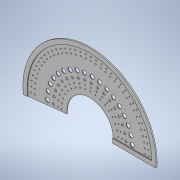
# Autodesk Inventor part: linerCone
Saved by Autodesk Inventor 2021.2 (Build 252289000, 289)
## iProperties
Created: 2021-06-06
Part Number: linerCone
Material: Generic
Document SubType Name: Modeling
Designer: Ryan
Density: 1 g/cm^3
Appearance: Default
Author: Ryan
Autodesk Inventor part; units mm, degrees
ref_plane "YZ Plane" through (0, 0, 0) normal (1, 0, 0) x (0, 1, 0)
ref_plane "XZ Plane" through (0, 0, 0) normal (0, 1, 0) x (-1, 0, 0)
ref_plane "XY Plane" through (0, 0, 0) normal (0, 0, 1) x (1, 0, 0)
sketch "Sketch1" plane through (0, 0, 0) normal (0, 0, 1) x (1, 0, 0)
  arc A0 (33.7972, 0) -> (-33.6117, -3.5367) centre (0, 0) ccw
  line L0 (0, 0) -> (-33.6117, -3.5367) construction
  line L1 (0, 0) -> (33.7972, 0) construction
  arc A1 (90.9472, 0) -> (-90.4486, -9.5105) centre (0, 0) ccw
  line L2 (0, 0) -> (-90.4486, -9.5105) construction
  line L3 (0, 0) -> (90.9472, 0) construction
  line L4 (33.7972, 0) -> (90.9472, 0)
  line L5 (-33.6117, -3.5367) -> (-90.4486, -9.5105)
  dimension "d2" = 33.7972
  dimension "d3" = 186.007
  dimension "d4" = 90.9472
  dimension "d5" = 186.002
  constraints: 12 end point, 4 point on circle, 2 centre point, 2 coincident, 1 collinear
  measures "d2" radius of A0
  measures "d4" radius of A1
extrude "Extrusion1" add sketch "Sketch1" along normal blind 0.7937
sketch "Sketch2" plane through (0, 0, 0.7937) normal (0, 0, 1) x (1, 0, 0)
  arc A0 (97.2972, 0) -> (-96.7638, -10.1743) centre (0, 0) ccw
  line L0 (-90.4486, -9.5105) -> (-33.6117, -3.5367) projected
  line L1 (-33.6117, -3.5367) -> (-96.7638, -10.1743)
  arc A1 (90.9472, 0) -> (-90.4486, -9.5105) centre (0, 0) ccw projected
  line L2 (33.7972, 0) -> (90.9472, 0) projected
  line L3 (33.7972, 0) -> (97.2972, 0)
  arc A2 (33.7972, 0) -> (-33.6117, -3.5367) centre (0, 0) ccw projected
  line L4 (33.7972, 0) -> (97.0898, 0)
  line L5 (97.0898, 0) -> (97.0898, -6.35)
  line L6 (97.0898, -6.35) -> (33.7972, -6.35)
  line L7 (33.7972, -6.35) -> (33.7972, 0)
  dimension "d10" = 97.2972
  dimension "d13" = 6.35
  constraints: 12 end point, 3 point on circle, 2 collinear, 2 parallel, 1 centre point, 1 coincident, 1 horizontal, 1 perpendicular
  measures "d10" radius of A0
  measures "d13" distance of L4.end L5.end
extrude "Extrusion2" add sketch "Sketch2" along normal mid plane 1.5875 contours L3 A1 L1 A0 | L5 L6 L7 L2 L3
sketch "Sketch3" plane through (0, 0, 0.7937) normal (0, 0, 1) x (1, 0, 0)
  circle A0 centre (80.7872, 2.54) radius 0.7938
  circle A1 centre (85.8672, 2.54) radius 0.7937
  line L0 (33.7972, 0) -> (33.7972, -6.35) projected
  line L1 (90.9472, 0) -> (33.7972, 0) projected
  point P0 (0, 0)
  dimension "d14" = 1.5875
  dimension "d15" = 1.5875
  dimension "d18" = 2.54
  dimension "d19" = 2.54
  dimension "d34" = 5.08
  dimension "d35" = 10.16
  constraints: 2 centre point, 1 coincident
  measures "d14" diameter of A0
  measures "d15" diameter of A1
  measures "d18" distance from line of L1 A0.centre
  measures "d19" distance from line of L1 A1.centre
  measures "d34" horizontal distance of point (90.947, 0) A1.centre
  measures "d35" horizontal distance of A0.centre L1.start
extrude "Extrusion3" cut sketch "Sketch3" against normal through all
pattern_circular "Circular Pattern1" count 36 over 180 about axis through (0, 0, 0) along (0, 0, 1) of "Extrusion3"
sketch "Sketch4" plane through (0, 0, 0.7937) normal (0, 0, 1) x (1, 0, 0)
  circle A0 centre (61.7372, 5.08) radius 3.175
  circle A1 centre (52.8472, 5.08) radius 1.5875
  circle A2 centre (46.4972, 5.08) radius 0.7938
  circle A3 centre (41.4172, 5.08) radius 0.7937
  line L0 (90.9472, 0) -> (33.7972, 0) projected
  line L1 (33.7972, 0) -> (33.7972, -6.35) projected
  circle A4 centre (80.7872, 2.54) radius 0.7938 projected
  point P0 (0, 0)
  dimension "d25" = 6.35
  dimension "d26" = 3.175
  dimension "d27" = 1.5875
  dimension "d28" = 1.5875
  dimension "d29" = 5.08
  dimension "d30" = 5.08
  dimension "d31" = 5.08
  dimension "d32" = 5.08
  dimension "d36" = 19.05
  dimension "d37" = 12.7
  dimension "d38" = 7.62
  dimension "d44" = 19.05
  constraints: 4 centre point, 1 coincident
  measures "d25" diameter of A0
  measures "d26" diameter of A1
  measures "d27" diameter of A2
  measures "d28" diameter of A3
  measures "d29" distance from line of L0 A0.centre
  measures "d30" distance from line of L0 A1.centre
  measures "d31" distance from line of L0 A2.centre
  measures "d32" distance from line of L0 A3.centre
  measures "d36" horizontal distance of A1.centre L0.end
  measures "d37" horizontal distance of L0.end A2.centre
  measures "d38" horizontal distance of L0.end A3.centre
  measures "d44" horizontal distance of A4.centre A0.centre
extrude "Extrusion4" cut sketch "Sketch4" against normal blind 1.5875 contours A0 | A1 | A2 | A3
pattern_circular "Circular Pattern2" count 18 over 175 about axis through (0, 0, 0) along (0, 0, 1) of "Extrusion4"
body "Solid1"
